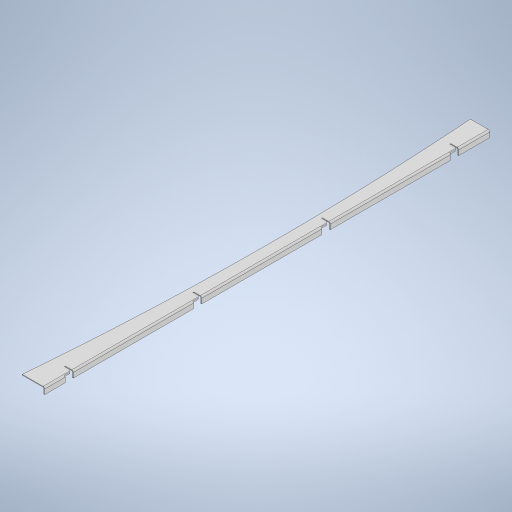
# Autodesk Inventor part: МОО 040 шпангоут борт 1
Saved by Autodesk Inventor 2024.2 (Build 282272000, 272)
## iProperties
Created: 2024-04-28
Part Number: МОО 040 шпангоут борт 1
Material: Generic
Document SubType Name: Sheet Metal
Designer: admin
Density: 1 g/cm^3
Sheet Metal Rule: Default_mm
Appearance: Default
Flat Pattern Width: 173.231 cm
Flat Pattern Length: 10.689 cm
Flat Pattern Area: 1851.66 cm^2
Sheet Metal Width: 1732,312 mm
Sheet Metal Length: 106,890 mm
Sheet Metal Area: 185166,018 mm^2
Стрингер_3: 67,157 mm
Стрингер_4: 48,106 mm
Стрингер_5: 51,700 mm
Стрингер_6: 77,959 mm
Author: admin
Autodesk Inventor part; units mm, degrees
ref_plane "YZ Plane" through (0, 0, 0) normal (1, 0, 0) x (0, 1, 0)
ref_plane "XZ Plane" through (0, 0, 0) normal (0, 1, 0) x (-1, 0, 0)
ref_plane "XY Plane" through (0, 0, 0) normal (0, 0, 1) x (1, 0, 0)
sketch "Sketch1" plane through (0, 0, 0) normal (0, 0, 1) x (1, 0, 0)
  arc A0 (750, -2100) -> (770.156, -238.4205) centre (-10250, -1050) ccw construction
  arc A1 (752.9864, -2100.2851) -> (771.2831, -213.263) centre (-10246.9891, -1050.0292) ccw
  line L0 (-750, -2700) -> (-750, 0) construction
  line L1 (-800, 50) -> (-800, -2750) construction
  line L2 (-850, -2800) -> (-850, 100) construction
  line L3 (850, 100) -> (850, -2800)
  line L4 (800, -2750) -> (800, 50) construction
  line L5 (750, 0) -> (750, -2700) construction
  line L6 (770.156, -238.4205) -> (767.1641, -238.6409) construction
  line L7 (768.2917, -213.4901) -> (771.2831, -213.263) construction
  arc A2 (747.4657, -5.0326) -> (744.8748, -2.3426) centre (744.4792, -5.3164) ccw construction
  arc A3 (747.4657, -5.0326) -> (747.0136, -0.2851) centre (-10252.9895, -1050.2527) ccw construction
  arc A4 (767.1641, -238.6409) -> (747.4657, -5.0326) centre (-10252.9895, -1050.2527) ccw construction
  line L8 (750, 0) -> (747.0136, -0.2851) construction
  arc A5 (750.4522, -4.7486) -> (750, 0) centre (-10250, -1050) ccw construction
  arc A6 (750.4522, -4.7486) -> (745.2706, 0.6314) centre (744.4791, -5.3162) ccw
  line L9 (-750, 0) -> (750, 0) construction
  line L10 (-850, 100) -> (850, 100) construction
  line L11 (800, 50) -> (-800, 50) construction
  arc A7 (770.156, -238.4205) -> (750.4522, -4.7486) centre (-10250, -1050) ccw
  line L12 (750, -2700) -> (-750, -2700) construction
  line L13 (750, -2100) -> (752.9864, -2100.2851) construction
  line L14 (-800, -2750) -> (800, -2750)
  line L15 (850, -2800) -> (-850, -2800) construction
  arc A8 (110, -2700) -> (114.1118, -2698.3696) centre (110, -2694) ccw construction
  line L16 (0, -2697) -> (110, -2697) construction
  line L17 (0, -2700) -> (0, -2697) construction
  arc A9 (750, 0) -> (745.2706, 0.6314) centre (0, -5600) ccw construction
  line L18 (750, 0) -> (749.6018, -2.9735) construction
  arc A10 (750, -3.0268) -> (0, 47) centre (-0.2, -5603) ccw construction
  line L19 (0, 47) -> (0, 0) construction
  line L20 (0, 50) -> (0, 47) construction
  line L21 (0, 100) -> (0, 50)
  arc A11 (745.2706, 0.6314) -> (0, 50) centre (0, -5600) ccw construction
  line L22 (-750, -2100) -> (750, -2100) construction
  arc A12 (110, -2697) -> (112.0559, -2696.1848) centre (110, -2694) ccw construction
  line L23 (676.3163, -2173.4556) -> (674.2605, -2171.2708) construction
  line L24 (690.4112, -2151.9536) -> (692.4671, -2154.1384) construction
  line L25 (752.0559, -2102.1848) -> (676.3163, -2173.4556) construction
  line L26 (114.1118, -2698.3696) -> (750, -2100) construction
  arc A13 (752.0559, -2102.1848) -> (752.9864, -2100.2851) centre (749.9998, -2099.9999) ccw construction
  line L27 (750, -2100) -> (752.0559, -2102.1848) construction
  arc A14 (749.1768, -2100.7746) -> (750.1074, -2098.8746) centre (747.1209, -2098.5898) ccw construction
  line L28 (112.0559, -2696.1848) -> (690.4112, -2151.9536) construction
  line L29 (850, -258.4205) -> (774.6194, -258.4205)
  arc A15 (800, 50) -> (0, 100) centre (0, -6325) ccw construction
  arc A16 (824.6194, -258.4205) -> (800, 50) centre (-10711.2413, -1024.069) ccw construction
  line L30 (824.6194, -258.4205) -> (824.6194, 100) construction
  arc A17 (789.8132, -2131.1922) -> (824.6194, -258.4205) centre (-10201.1223, -990.2118) ccw construction
  line L31 (0, -2700) -> (0, -2750) construction
  line L32 (112.3791, -2700) -> (132.2053, -2750) construction
  line L33 (132.2053, -2750) -> (850, -2074.5565)
  arc A18 (770.0996, -238.4247) -> (766.3709, -188.564) centre (768.2917, -213.4901) ccw construction
  line L34 (850, -400) -> (783.8749, -400) construction
  line L35 (850, -900) -> (801.9923, -900) construction
  line L36 (850, -1400) -> (797.4674, -1400) construction
  line L37 (850, -1900) -> (770.2723, -1900) construction
  line L38 (350, 100) -> (350, 39.1489)
  line L39 (-1472.612, -150) -> (-973.4947, -150)
  line L40 (-1472.612, -700) -> (-973.4947, -700)
  line L41 (-1472.612, -1250) -> (-973.4947, -1250)
  line L42 (-1472.612, -1800) -> (-973.4947, -1800)
  line L43 (800, -2750) -> (850, -2750) construction
  line L44 (762.8963, -1990.7324) -> (850, -1990.7324)
  dimension "d16" = 1500
  dimension "d17" = 2700
  dimension "d18" = 2100
  dimension "d19" = 6
  dimension "d20" = 3
  dimension "d21" = 3
  dimension "d22" = 6
  dimension "d23" = 3
  dimension "d24" = 239.271
  dimension "d25" = 50
  dimension "d26" = 50
  dimension "d27" = 3
  dimension "d28" = 110
  dimension "d29" = 25
  dimension "d30" = 104
  dimension "d31" = 25
  dimension "d32" = 20
  dimension "d33" = 50
  dimension "d57" = 500
  dimension "d58" = 500
  dimension "d59" = 500
  dimension "d60" = 500
  dimension "d61" = 500
  dimension "d83" = 250
  dimension "d86" = 550
  dimension "d91" = 274.5565
  dimension "d103" = 110
  measures "d16" distance of L0.end L5.start
  measures "d17" distance of L5.start L5.end
  measures "d18" distance between parallel lines of L22 L9
  measures "d19" radius of A6
  measures "d20" radius of A2
  measures "d21" radius of A14
  measures "d22" radius of A8
  measures "d23" radius of A12
  measures "d24" distance of L6.start L5.start
  measures "d25" distance between parallel lines of L11 L10
  measures "d26" distance between parallel lines of L9 L11
  measures "d27" distance of L21.end L19.start
  measures "d28" distance from line of L17 A8.centre
  measures "d29" distance of L23.end L24.end
  measures "d30" distance of L27.start L23.end
  measures "d31" distance of L6.start L7.start
  measures "d32" vertical distance of L6.start L29.end
  measures "d33" distance of L30.start L29.end
  measures "d57" distance between parallel lines of L34 L10
  measures "d58" distance between parallel lines of L35 L34
  measures "d59" distance between parallel lines of L35 L36
  measures "d60" distance between parallel lines of L36 L37
  measures "d83" distance between parallel lines of L39 L10
  measures "d86" distance of L39.start L40.start
  measures "d91" distance from line of L33.end L42
  measures "d103" distance of L44.start L13.end
extrude "Plate3" add sketch "Sketch1" along normal blind 3
sketch "Sketch3" plane through (847, -258.4205, 3) normal (1, 0, 0) x (0, 1, 0)
  line L0 (-1732.3118, 0) -> (0, 0)
  line L1 (0, 0) -> (0, 25)
  line L2 (0, 25) -> (-1732.3118, 25)
  line L3 (-1732.3118, 25) -> (-1732.3118, 0)
  constraints: 6 end point, 1 horizontal, 1 perpendicular, 1 vertical
edge flange "Flange2" height 25 angle 90 thickness 3 bend radius 3 thickness toward (1, 0, 0) relief straight relief width 3 relief depth 1.5 edges at (850, -1124.5764, 3) wall of the first edge with corners at (847, -1990.7324, 3) (847, -258.4205, 3) (847, -258.4205, -22) (847, -1990.7324, -22)
bend "Bend2"
corner "Corner2"
sketch "Sketch5" plane through (0, 0, 0) normal (0, 0, 1) x (1, 0, 0)
  line L0 (844, -1990.7324) -> (844, -258.4205) projected
  line L1 (774.6194, -258.4205) -> (844, -258.4205) projected
  arc A0 (762.8963, -1990.7324) -> (774.6194, -258.4205) centre (-10246.9891, -1050.0292) ccw projected
  line L2 (850, -258.4205) -> (850, -1990.7324) projected
  line L3 (850, -379.4205) -> (782.6429, -379.4205)
  line L4 (850, -382.4205) -> (782.8249, -382.4205)
  line L5 (847, -1990.7324) -> (847, -258.4205) projected
  line L6 (819, -379.4205) -> (819, -382.4205)
  line L7 (844, -411.4205) -> (850, -411.4205)
  line L8 (850, -879.4205) -> (801.6937, -879.4205)
  line L9 (850, -882.4205) -> (801.7396, -882.4205)
  line L10 (819, -879.4205) -> (819, -882.4205)
  line L11 (850, -1379.4205) -> (798.1003, -1379.4205)
  line L12 (850, -1382.4205) -> (798.0104, -1382.4205)
  line L13 (819, -1379.4205) -> (819, -1382.4205)
  line L14 (850, -1879.4205) -> (771.8406, -1879.4205)
  line L15 (850, -1882.4205) -> (771.6144, -1882.4205)
  line L16 (819, -1879.4205) -> (819, -1882.4205)
  line L17 (850, -911.4205) -> (844, -911.4205)
  line L18 (844, -1411.4205) -> (850, -1411.4205)
  line L19 (844, -1911.4205) -> (850, -1911.4205)
  line L20 (844, -1990.7324) -> (762.8963, -1990.7324) projected
  point P0 (0, 0)
  point P1 (844, -382.4205)
  point P2 (847, -382.4205)
  point P3 (847, -411.4205)
  point P4 (847, -1911.4205)
  point P5 (847, -1882.4205)
  point P6 (847, -1411.4205)
  point P7 (847, -1382.4205)
  point P8 (847, -911.4205)
  point P9 (847, -882.4205)
  dimension "d69" = 1732.3118
  dimension "d70" = 3
  dimension "d76" = 67.3571
  dimension "d77" = 31
  dimension "d78" = 121
  dimension "d79" = 32
  dimension "d80" = 48.3063
  dimension "d81" = 31
  dimension "d82" = 500
  dimension "d92" = 500
  dimension "d93" = 500
  dimension "d94" = 32
  dimension "d95" = 31
  dimension "d96" = 32
  dimension "d97" = 31
  dimension "d98" = 32
  dimension "d102" = 78.1594
  dimension "d104" = 51.8997
  constraints: 32 end point, 12 point on line, 7 horizontal, 7 perpendicular, 3 collinear, 3 parallel, 22 other
  measures "d69" distance of point (850, -258.421) point (850, -1990.732)
  measures "d70" distance between parallel lines of L4 L3
  measures "d76" distance of L3.start L3.end
  measures "d78" distance from line of L3 L5.end
  measures "d79" distance between parallel lines of L7 L3
  measures "d80" distance of L8.start L8.end
  measures "d82" distance between parallel lines of L8 L3
  measures "d92" distance between parallel lines of L11 L8
  measures "d93" distance between parallel lines of L14 L11
  measures "d94" distance of L17.start L8.start
  measures "d95" distance of L13.start L11.start
  measures "d96" distance of L18.end L11.start
  measures "d97" distance of L16.start L14.start
  measures "d98" distance of L19.end L14.start
  measures "d102" distance of L14.start L14.end
  measures "d104" distance of L11.end L11.start
extrude "Extrusion2" cut sketch "Sketch5" along normal through all both and the other way through all contours L6 L3 L0 L4 | L0 L3 L5 L4 | L5 L4 L2 L7 | L5 L3 L2 L4
chamfer "Chamfer1" distance 8 angle 45 1 edges at (847, -382.4205, -0.4019)
pattern_linear "Rectangular Pattern2" count 4 spacing 500 along (0, -1, 0) of "Extrusion2", "Chamfer1"
equation "\"d16\" = d34"
equation "\"d17\" = d35"
equation "\"d18\" = d36"
equation "\"d19\" = d37"
equation "\"d20\" = d38"
equation "\"d21\" = d39"
equation "\"d22\" = d39 + d43"
equation "\"d23\" = d39"
equation "\"d24\" = d40"
equation "\"d27\" = d39"
equation "\"d28\" = 0.5 * d44"
equation "\"d29\" = d41"
equation "\"d30\" = d42"
equation "\"d31\" = d41"
equation "\"d33\" = d25"
equation "\"BendRadius\" = Thickness"
equation "\"BendReliefWidth\" = Thickness"
equation "\"BendReliefDepth\" = 0.5 * Thickness"
equation "\"CornerReliefSize\" = 4 * Thickness"
equation "\"MinimumRemnant\" = 2 * Thickness"
equation "\"TransitionRadius\" = BendRadius"
equation "\"JacobiRadiusSize\" = BendRadius"
equation "\"GapSize\" = Thickness"
equation "\"Стрингер_3\" = 67.15706"
equation "\"d37\" = d39 + d43"
equation "\"d38\" = d39"
equation "\"d43\" = d39"
equation "\"Стрингер_4\" = 48.1063"
equation "\"Стрингер_5\" = 51.69968"
equation "\"Стрингер_6\" = 77.95935"
equation "\"d34\" = 1500"
equation "\"d35\" = 2700"
equation "\"d36\" = 2100"
equation "\"d39\" = 3"
equation "\"d40\" = 239.271"
equation "\"d44\" = 220"
equation "\"d41\" = 25"
equation "\"d42\" = 104"
equation "\"Thickness\" = 3"
body "Solid2"
